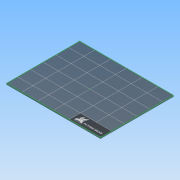
# Autodesk Inventor part: ультрабаза
Saved by Autodesk Inventor 2017 (Build 210142000, 142)
## iProperties
Part Number: ультрабаза
Material: Типовые
Document SubType Name: Modeling
Designer: Max
Mass: 234.623 g
Surface Area: 1209.8 cm^2
Volume: 234.623 cm^3
Density: 1 g/cm^3
Appearance: Металлическая сетка 01
Author: Max
Autodesk Inventor part; units mm, degrees
(part 1 of 2)
ref_plane "YZ Plane" through (0, 0, 0) normal (1, 0, 0) x (0, 1, 0)
ref_plane "XZ Plane" through (0, 0, 0) normal (0, 1, 0) x (-1, 0, 0)
ref_plane "XY Plane" through (0, 0, 0) normal (0, 0, 1) x (1, 0, 0)
sketch "Эскиз1" plane through (0, 0, 0) normal (0, 0, 1) x (1, 0, 0)
  line L0 (135.5, -107) -> (-135.5, -107)
  line L1 (-137.5, -105) -> (-137.5, 105)
  line L2 (-135.5, 107) -> (135.5, 107)
  line L3 (137.5, 105) -> (137.5, -105)
  line L4 (137.5, -107) -> (-137.5, 107) construction
  line L5 (-137.5, -107) -> (137.5, 107) construction
  arc A0 (-135.5, 107) -> (-137.5, 105) centre (-135.5, 105) ccw
  arc A1 (137.5, 105) -> (135.5, 107) centre (135.5, 105) ccw
  arc A2 (135.5, -107) -> (137.5, -105) centre (135.5, -105) ccw
  arc A3 (-137.5, -105) -> (-135.5, -107) centre (-135.5, -105) ccw
  point P0 (0, 0)
  dimension "d0" = 214
  dimension "d1" = 275
  dimension "d2" = 2
  constraints: 12 end point, 8 point on circle, 8 point on line, 8 tangent, 4 centre point, 3 equal radius, 2 midpoint, 2 parallel, 1 horizontal, 1 perpendicular
  measures "d0" distance between parallel lines of L0 L2
  measures "d1" distance between parallel lines of L3 L1
  measures "d2" radius of A0
extrude "Выдавливание1" add sketch "Эскиз1" along normal blind 4
chamfer "Фаска1" distance 1 angle 45 16 edges at (137.5, 0, 4) (136.9142, 106.4142, 4) (0, 107, 4) (-136.9142, 106.4142, 4) (-137.5, 0, 4) (-136.9142, -106.4142, 4) (0, -107, 4) (136.9142, -106.4142, 4) (137.5, 0, 0) (136.9142, 106.4142, 0) (0, 107, 0) (-136.9142, 106.4142, 0) (-137.5, 0, 0) (-136.9142, -106.4142, 0) (0, -107, 0) (136.9142, -106.4142, 0)
sketch "Эскиз2" plane through (0, 0, 4) normal (0, 0, 1) x (1, 0, 0)
  line L0 (136.5, 105) -> (136.5, -105) projected
  arc A0 (136.5, 105) -> (135.5, 106) centre (135.5, 105) ccw projected
  line L1 (-135.5, 106) -> (135.5, 106) projected
  arc A1 (-135.5, 106) -> (-136.5, 105) centre (-135.5, 105) ccw projected
  line L2 (-136.5, -105) -> (-136.5, 105) projected
  arc A2 (-136.5, -105) -> (-135.5, -106) centre (-135.5, -105) ccw projected
  line L3 (135.5, -106) -> (-135.5, -106) projected
  arc A3 (135.5, -106) -> (136.5, -105) centre (135.5, -105) ccw projected
  point P0 (0, 0)
sketch "Эскиз3" plane through (0, 0, 4) normal (0, 0, 1) x (1, 0, 0)
  line L0 (-136.5, -105) -> (-136.5, 105) projected
  line L1 (136.5, 105) -> (136.5, -105) projected
  line L2 (-136.5, 0.35) -> (136.5, 0.35)
  line L3 (136.5, 0.35) -> (136.5, -0.35)
  line L4 (136.5, -0.35) -> (-136.5, -0.35)
  line L5 (-136.5, -0.35) -> (-136.5, 0.35)
  line L6 (0, 0) -> (33.6599, 0) construction
  line L7 (0, 0) -> (0, 3.0622)
  line L8 (0, 3.0622) -> (0, 34.6111) construction
  line L9 (135.5, -106) -> (-135.5, -106) projected
  line L10 (-135.5, 106) -> (135.5, 106) projected
  line L11 (-0.35, -106) -> (0.35, -106)
  line L12 (0.35, -106) -> (0.35, 106)
  line L13 (0.35, 106) -> (-0.35, 106)
  line L14 (-0.35, 106) -> (-0.35, -106)
  dimension "d8" = 0.7
  dimension "d17" = 0.7
  constraints: 22 end point, 5 parallel, 5 point on line, 2 horizontal, 2 perpendicular, 2 other
  measures "d8" distance between parallel lines of L4 L2
  measures "d17" distance between parallel lines of L12 L14
extrude "Выдавливание2" add sketch "Эскиз3" along normal blind 0.1 contours L0 L2 L14 L4 | L14 L2 L12 L4 | L12 L2 L1 L4
pattern_linear "Прямоуг.массив1" count 3 spacing 37 along (0, 1, 0) count 3 spacing 37 along (0, -1, 0) of "Выдавливание2"
extrude "Выдавливание3" add sketch "Эскиз3" along normal blind 0.1 contours L14 L2 L12 L4 | L4 L12 L9 L14 | L14 L10 L12 L2
pattern_linear "Прямоуг.массив2" count 3 spacing 46 along (-1, 0, 0) count 3 spacing 46 along (1, 0, 0) of "Выдавливание3"
sketch "Эскиз4" plane through (0, 0, 4.1) normal (0, 0, 1) x (1, 0, 0)
  line L0 (-135.5, -106) -> (135.5, -106) projected
  line L1 (91.65, -74.35) -> (92.35, -74.35)
  line L2 (92.35, -74.35) -> (92.35, -106)
  line L3 (92.35, -106) -> (91.65, -106)
  line L4 (91.65, -106) -> (91.65, -74.35)
  line L5 (92.35, -106) -> (92.35, -74.35) projected
  point P0 (0, 0)
  constraints: 8 end point, 2 parallel, 1 collinear, 1 horizontal, 1 perpendicular, 1 point on line
extrude "Выдавливание4" cut sketch "Эскиз4" against normal blind 0.1
sketch "Эскиз6" plane through (0, 0, 4) normal (0, 0, 1) x (1, 0, 0)
  line L0 (47.8519, -76.7152) -> (78.2896, -76.7152) construction
  line L1 (78.2896, -76.7152) -> (78.2896, -107.153) construction
  line L2 (78.2896, -107.153) -> (47.8519, -107.153) construction
  line L3 (47.8519, -107.153) -> (47.8519, -76.7152) construction
  line L4 (58.0569, -84.1432) -> (58.585, -83.5976) construction
  line L5 (58.585, -83.5976) -> (59.2465, -82.9077) construction
  line L6 (59.2465, -82.9077) -> (59.6838, -82.432) construction
  line L7 (59.6838, -82.432) -> (59.9462, -82.0822) construction
  line L8 (59.9462, -82.0822) -> (60.5989, -81.4036) construction
  line L9 (60.5989, -81.4036) -> (61.1809, -80.7023) construction
  line L10 (61.1809, -80.7023) -> (61.3763, -80.4637) construction
  line L11 (61.3763, -80.4637) -> (62.6475, -78.5746) construction
  line L12 (62.6475, -78.5746) -> (62.8189, -78.3137) construction
  line L13 (62.8189, -78.3137) -> (63.1024, -77.7856) construction
  line L14 (63.1024, -77.7856) -> (63.3659, -77.2628) construction
  line L15 (63.3659, -77.2628) -> (63.6158, -76.7664) construction
  line L16 (63.6158, -76.7664) -> (63.6201, -76.7558) construction
  line L17 (63.6201, -76.7558) -> (63.6201, -76.7654) construction
  line L18 (63.6201, -76.7654) -> (63.7564, -77.0283) construction
  line L19 (63.7564, -77.0283) -> (64.02, -77.8831) construction
  line L20 (64.02, -77.8831) -> (64.0864, -78.3234) construction
  line L21 (64.0864, -78.3234) -> (64.0864, -78.7811) construction
  line L22 (64.0864, -78.7811) -> (63.9126, -80.1417) construction
  line L23 (63.9126, -80.1417) -> (63.6859, -80.7747) construction
  line L24 (63.6859, -80.7747) -> (63.2325, -81.8429) construction
  line L25 (63.2325, -81.8429) -> (62.816, -82.539) construction
  line L26 (62.816, -82.539) -> (62.3595, -83.2522) construction
  line L27 (62.3595, -83.2522) -> (62.2397, -83.4291) construction
  line L28 (62.2397, -83.4291) -> (62.0693, -83.676) construction
  line L29 (62.0693, -83.676) -> (62.1075, -83.6534) construction
  line L30 (62.1075, -83.6534) -> (62.1613, -83.6199) construction
  line L31 (62.1613, -83.6199) -> (62.3249, -83.4891) construction
  line L32 (62.3249, -83.4891) -> (62.9319, -82.8314) construction
  line L33 (62.9319, -82.8314) -> (63.8264, -81.7452) construction
  line L34 (63.8264, -81.7452) -> (64.8316, -80.3842) construction
  line L35 (64.8316, -80.3842) -> (64.8415, -80.3689) construction
  line L36 (64.8415, -80.3689) -> (64.836, -80.3846) construction
  line L37 (64.836, -80.3846) -> (64.8649, -80.4981) construction
  line L38 (64.8649, -80.4981) -> (64.9349, -80.9101) construction
  line L39 (64.9349, -80.9101) -> (65.0014, -81.5135) construction
  line L40 (65.0014, -81.5135) -> (64.9087, -82.4789) construction
  line L41 (64.9087, -82.4789) -> (64.606, -83.4734) construction
  line L42 (64.606, -83.4734) -> (64.1613, -84.3443) construction
  line L43 (64.1613, -84.3443) -> (63.6672, -85.1103) construction
  line L44 (63.6672, -85.1103) -> (62.9587, -85.9145) construction
  line L45 (62.9587, -85.9145) -> (62.6125, -86.2444) construction
  line L46 (62.6125, -86.2444) -> (62.3243, -86.521) construction
  line L47 (62.3243, -86.521) -> (62.171, -86.686) construction
  line L48 (62.171, -86.686) -> (62.162, -86.6995) construction
  line L49 (62.162, -86.6995) -> (62.1856, -86.6864) construction
  line L50 (62.1856, -86.6864) -> (62.4487, -86.5194) construction
  line L51 (62.4487, -86.5194) -> (62.7136, -86.3821) construction
  line L52 (62.7136, -86.3821) -> (63.2176, -86.0665) construction
  line L53 (63.2176, -86.0665) -> (63.723, -85.7352) construction
  line L54 (63.723, -85.7352) -> (64.0161, -85.4507) construction
  line L55 (64.0161, -85.4507) -> (64.3389, -85.1406) construction
  line L56 (64.3389, -85.1406) -> (64.5597, -84.9113) construction
  line L57 (64.5597, -84.9113) -> (64.5708, -84.896) construction
  line L58 (64.5708, -84.896) -> (64.5656, -84.9151) construction
  line L59 (64.5656, -84.9151) -> (64.6262, -85.2714) construction
  line L60 (64.6262, -85.2714) -> (64.5771, -85.7127) construction
  line L61 (64.5771, -85.7127) -> (64.1613, -87.1292) construction
  line L62 (64.1613, -87.1292) -> (63.5106, -88.2303) construction
  line L63 (63.5106, -88.2303) -> (62.3182, -89.6027) construction
  line L64 (62.3182, -89.6027) -> (62.3174, -89.6036) construction
  line L65 (62.3174, -89.6036) -> (62.32, -89.6029) construction
  line L66 (62.32, -89.6029) -> (62.9995, -89.5699) construction
  line L67 (62.9995, -89.5699) -> (63.0073, -89.5699) construction
  line L68 (63.0073, -89.5699) -> (63.0203, -89.5624) construction
  line L69 (63.0203, -89.5624) -> (63.3181, -89.4088) construction
  line L70 (63.3181, -89.4088) -> (63.7593, -89.0384) construction
  line L71 (63.7593, -89.0384) -> (64.1508, -88.6371) construction
  line L72 (64.1508, -88.6371) -> (64.5553, -88.1503) construction
  line L73 (64.5553, -88.1503) -> (64.9848, -87.3865) construction
  line L74 (64.9848, -87.3865) -> (65.1279, -86.9947) construction
  line L75 (65.1279, -86.9947) -> (65.3006, -86.2605) construction
  line L76 (65.3006, -86.2605) -> (65.3006, -85.8673) construction
  line L77 (65.3006, -85.8673) -> (65.3006, -85.207) construction
  line L78 (65.3006, -85.207) -> (65.1992, -84.7863) construction
  line L79 (65.1992, -84.7863) -> (65.0979, -84.5614) construction
  line L80 (65.0979, -84.5614) -> (64.9939, -84.3167) construction
  line L81 (64.9939, -84.3167) -> (64.9664, -84.1432) construction
  line L82 (64.9664, -84.1432) -> (64.9922, -83.8019) construction
  line L83 (64.9922, -83.8019) -> (65.1313, -83.509) construction
  line L84 (65.1313, -83.509) -> (65.3023, -83.2527) construction
  line L85 (65.3023, -83.2527) -> (65.74, -82.8881) construction
  line L86 (65.74, -82.8881) -> (66.2485, -82.5981) construction
  line L87 (66.2485, -82.5981) -> (67.1006, -82.2368) construction
  line L88 (67.1006, -82.2368) -> (68.0195, -81.8844) construction
  line L89 (68.0195, -81.8844) -> (69.5796, -81.1161) construction
  line L90 (69.5796, -81.1161) -> (71.2261, -80.3458) construction
  line L91 (71.2261, -80.3458) -> (72.7714, -79.4408) construction
  line L92 (72.7714, -79.4408) -> (73.5994, -78.8823) construction
  line L93 (73.5994, -78.8823) -> (75.316, -77.7088) construction
  line L94 (75.316, -77.7088) -> (75.8413, -77.2797) construction
  line L95 (75.8413, -77.2797) -> (76.1159, -77.0359) construction
  line L96 (76.1159, -77.0359) -> (76.2395, -76.9192) construction
  line L97 (76.2395, -76.9192) -> (76.2524, -76.9192) construction
  line L98 (76.2524, -76.9192) -> (76.2201, -77.0074) construction
  line L99 (76.2201, -77.0074) -> (76.2201, -77.2657) construction
  line L100 (76.2201, -77.2657) -> (76.1001, -77.9758) construction
  line L101 (76.1001, -77.9758) -> (75.8421, -78.9571) construction
  line L102 (75.8421, -78.9571) -> (75.5423, -79.5608) construction
  line L103 (75.5423, -79.5608) -> (75.0505, -80.2964) construction
  line L104 (75.0505, -80.2964) -> (74.6067, -80.8242) construction
  line L105 (74.6067, -80.8242) -> (73.3049, -82.0792) construction
  line L106 (73.3049, -82.0792) -> (72.4409, -82.7407) construction
  line L107 (72.4409, -82.7407) -> (71.1828, -83.5927) construction
  line L108 (71.1828, -83.5927) -> (70.7434, -83.8471) construction
  line L109 (70.7434, -83.8471) -> (70.7434, -83.8614) construction
  line L110 (70.7434, -83.8614) -> (70.8232, -83.9129) construction
  line L111 (70.8232, -83.9129) -> (70.9595, -83.8861) construction
  line L112 (70.9595, -83.8861) -> (71.9932, -83.4155) construction
  line L113 (71.9932, -83.4155) -> (73.7755, -82.4723) construction
  line L114 (73.7755, -82.4723) -> (74.7969, -81.873) construction
  line L115 (74.7969, -81.873) -> (75.4744, -81.4665) construction
  line L116 (75.4744, -81.4665) -> (75.4973, -81.4518) construction
  line L117 (75.4973, -81.4518) -> (75.4973, -81.5379) construction
  line L118 (75.4973, -81.5379) -> (75.2536, -82.3724) construction
  line L119 (75.2536, -82.3724) -> (74.3062, -83.9127) construction
  line L120 (74.3062, -83.9127) -> (73.7236, -84.5338) construction
  line L121 (73.7236, -84.5338) -> (72.7954, -85.3581) construction
  line L122 (72.7954, -85.3581) -> (72.0406, -85.8668) construction
  line L123 (72.0406, -85.8668) -> (71.0807, -86.4494) construction
  line L124 (71.0807, -86.4494) -> (70.1289, -86.8842) construction
  line L125 (70.1289, -86.8842) -> (69.3987, -87.2042) construction
  line L126 (69.3987, -87.2042) -> (69.1115, -87.2616) construction
  line L127 (69.1115, -87.2616) -> (69.0889, -87.306) construction
  line L128 (69.0889, -87.306) -> (69.1488, -87.3298) construction
  line L129 (69.1488, -87.3298) -> (70.1619, -87.2655) construction
  line L130 (70.1619, -87.2655) -> (71.1536, -87.0008) construction
  line L131 (71.1536, -87.0008) -> (71.7613, -86.7659) construction
  line L132 (71.7613, -86.7659) -> (72.5321, -86.4474) construction
  line L133 (72.5321, -86.4474) -> (72.6124, -86.4147) construction
  line L134 (72.6124, -86.4147) -> (72.5643, -86.4496) construction
  line L135 (72.5643, -86.4496) -> (72.4297, -86.7091) construction
  line L136 (72.4297, -86.7091) -> (72.0429, -87.336) construction
  line L137 (72.0429, -87.336) -> (71.7462, -87.7207) construction
  line L138 (71.7462, -87.7207) -> (71.1519, -88.3518) construction
  line L139 (71.1519, -88.3518) -> (70.3788, -89.0405) construction
  line L140 (70.3788, -89.0405) -> (69.6666, -89.4997) construction
  line L141 (69.6666, -89.4997) -> (68.9778, -89.9073) construction
  line L142 (68.9778, -89.9073) -> (68.7389, -90.0573) construction
  line L143 (68.7389, -90.0573) -> (68.7212, -90.0868) construction
  line L144 (68.7212, -90.0868) -> (68.9979, -90.0868) construction
  line L145 (68.9979, -90.0868) -> (69.6455, -90.1548) construction
  line L146 (69.6455, -90.1548) -> (70.6365, -90.3216) construction
  line L147 (70.6365, -90.3216) -> (70.8988, -90.3216) construction
  line L148 (70.8988, -90.3216) -> (72.8573, -91.6694) construction
  line L149 (72.8573, -91.6694) -> (72.8654, -91.6787) construction
  line L150 (72.8654, -91.6787) -> (72.8941, -91.7359) construction
  line L151 (72.8941, -91.7359) -> (73.23, -92.4126) construction
  line L152 (73.23, -92.4126) -> (73.23, -92.496) construction
  line L153 (73.23, -92.496) -> (73.163, -92.7094) construction
  line L154 (73.163, -92.7094) -> (73.0011, -93.1785) construction
  line L155 (73.0011, -93.1785) -> (72.8815, -93.3901) construction
  line L156 (72.8815, -93.3901) -> (72.83, -93.403) construction
  line L157 (72.83, -93.403) -> (72.83, -93.3828) construction
  line L158 (72.83, -93.3828) -> (72.83, -93.3036) construction
  line L159 (72.83, -93.3036) -> (72.8116, -93.0902) construction
  line L160 (72.8116, -93.0902) -> (72.7674, -92.8952) construction
  line L161 (72.7674, -92.8952) -> (72.6515, -92.577) construction
  line L162 (72.6515, -92.577) -> (72.3701, -92.3194) construction
  line L163 (72.3701, -92.3194) -> (72.1033, -92.0876) construction
  line L164 (72.1033, -92.0876) -> (71.9782, -92.0379) construction
  line L165 (71.9782, -92.0379) -> (71.9285, -92.025) construction
  line L166 (71.9285, -92.025) -> (71.946, -92.0337) construction
  line L167 (71.946, -92.0337) -> (72.0417, -92.1122) construction
  line L168 (72.0417, -92.1122) -> (72.2698, -92.3774) construction
  line L169 (72.2698, -92.3774) -> (72.5703, -92.7673) construction
  line L170 (72.5703, -92.7673) -> (72.6719, -93.0395) construction
  line L171 (72.6719, -93.0395) -> (72.7693, -93.4294) construction
  line L172 (72.7693, -93.4294) -> (72.7693, -93.5984) construction
  line L173 (72.7693, -93.5984) -> (72.7693, -94.6006) construction
  line L174 (72.7693, -94.6006) -> (72.7693, -94.721) construction
  line L175 (72.7693, -94.721) -> (73.012, -95.0062) construction
  line L176 (73.012, -95.0062) -> (73.6685, -95.948) construction
  line L177 (73.6685, -95.948) -> (73.7068, -96.0386) construction
  line L178 (73.7068, -96.0386) -> (73.7068, -96.2499) construction
  line L179 (73.7068, -96.2499) -> (74.0406, -97.4838) construction
  line L180 (74.0406, -97.4838) -> (74.0406, -97.6417) construction
  line L181 (74.0406, -97.6417) -> (74.0046, -97.9554) construction
  line L182 (74.0046, -97.9554) -> (73.7015, -99.536) construction
  line L183 (73.7015, -99.536) -> (73.673, -99.536) construction
  line L184 (73.673, -99.536) -> (73.5426, -99.536) construction
  line L185 (73.5426, -99.536) -> (72.5119, -99.536) construction
  line L186 (72.5119, -99.536) -> (72.4208, -99.536) construction
  line L187 (72.4208, -99.536) -> (72.2665, -99.2589) construction
  line L188 (72.2665, -99.2589) -> (71.6001, -98.5264) construction
  line L189 (71.6001, -98.5264) -> (71.4238, -98.2675) construction
  line L190 (71.4238, -98.2675) -> (70.4213, -96.7197) construction
  line L191 (70.4213, -96.7197) -> (70.3885, -96.6426) construction
  line L192 (70.3885, -96.6426) -> (70.3113, -96.6216) construction
  line L193 (70.3113, -96.6216) -> (67.9932, -95.6736) construction
  line L194 (67.9932, -95.6736) -> (67.977, -95.6736) construction
  line L195 (67.977, -95.6736) -> (67.977, -95.7933) construction
  line L196 (67.977, -95.7933) -> (70.1244, -96.8272) construction
  line L197 (70.1244, -96.8272) -> (70.2246, -96.9143) construction
  line L198 (70.2246, -96.9143) -> (70.4218, -97.1682) construction
  line L199 (70.4218, -97.1682) -> (71.2221, -98.1928) construction
  line L200 (71.2221, -98.1928) -> (71.4717, -98.5349) construction
  line L201 (71.4717, -98.5349) -> (71.4717, -98.7274) construction
  line L202 (71.4717, -98.7274) -> (71.1015, -98.9495) construction
  line L203 (71.1015, -98.9495) -> (70.8349, -98.9495) construction
  line L204 (70.8349, -98.9495) -> (70.1833, -98.7669) construction
  line L205 (70.1833, -98.7669) -> (69.2694, -98.5446) construction
  line L206 (69.2694, -98.5446) -> (68.5464, -98.0323) construction
  line L207 (68.5464, -98.0323) -> (67.1489, -97.0367) construction
  line L208 (67.1489, -97.0367) -> (66.0385, -96.137) construction
  line L209 (66.0385, -96.137) -> (66.07, -96.1214) construction
  line L210 (66.07, -96.1214) -> (65.9547, -96.2124) construction
  line L211 (65.9547, -96.2124) -> (64.6537, -96.8644) construction
  line L212 (64.6537, -96.8644) -> (64.5984, -96.8644) construction
  line L213 (64.5984, -96.8644) -> (64.3032, -96.8644) construction
  line L214 (64.3032, -96.8644) -> (62.2656, -96.8644) construction
  line L215 (62.2656, -96.8644) -> (62.2288, -96.8561) construction
  line L216 (62.2288, -96.8561) -> (62.1845, -96.8167) construction
  line L217 (62.1845, -96.8167) -> (60.8689, -96.2809) construction
  line L218 (60.8689, -96.2809) -> (60.8266, -96.2809) construction
  line L219 (60.8266, -96.2809) -> (60.6629, -96.4775) construction
  line L220 (60.6629, -96.4775) -> (58.7049, -98.0118) construction
  line L221 (58.7049, -98.0118) -> (58.6154, -98.0651) construction
  line L222 (58.6154, -98.0651) -> (57.6146, -98.3598) construction
  line L223 (57.6146, -98.3598) -> (56.0021, -98.9381) construction
  line L224 (56.0021, -98.9381) -> (55.7852, -98.9715) construction
  line L225 (55.7852, -98.9715) -> (55.4405, -98.8492) construction
  line L226 (55.4405, -98.8492) -> (55.0624, -98.6823) construction
  line L227 (55.0624, -98.6823) -> (55.0624, -98.6656) construction
  line L228 (55.0624, -98.6656) -> (55.1681, -98.6088) construction
  line L229 (55.1681, -98.6088) -> (56.837, -97.1126) construction
  line L230 (56.837, -97.1126) -> (56.8672, -97.0916) construction
  line L231 (56.8672, -97.0916) -> (56.9191, -96.9557) construction
  line L232 (56.9191, -96.9557) -> (57.4616, -96.0024) construction
  line L233 (57.4616, -96.0024) -> (57.4616, -95.9863) construction
  line L234 (57.4616, -95.9863) -> (57.2446, -95.8979) construction
  line L235 (57.2446, -95.8979) -> (57.1964, -95.9519) construction
  line L236 (57.1964, -95.9519) -> (56.6746, -97.0084) construction
  line L237 (56.6746, -97.0084) -> (56.6189, -97.0976) construction
  line L238 (56.6189, -97.0976) -> (54.7059, -98.7912) construction
  line L239 (54.7059, -98.7912) -> (54.588, -98.8386) construction
  line L240 (54.588, -98.8386) -> (54.1498, -98.8386) construction
  line L241 (54.1498, -98.8386) -> (53.7434, -98.7814) construction
  line L242 (53.7434, -98.7814) -> (53.1643, -98.6693) construction
  line L243 (53.1643, -98.6693) -> (52.9154, -98.3774) construction
  line L244 (52.9154, -98.3774) -> (52.9154, -98.2185) construction
  line L245 (52.9154, -98.2185) -> (53.0184, -98.0297) construction
  line L246 (53.0184, -98.0297) -> (53.4219, -97.7635) construction
  line L247 (53.4219, -97.7635) -> (53.7439, -97.6862) construction
  line L248 (53.7439, -97.6862) -> (54.1302, -97.4544) construction
  line L249 (54.1302, -97.4544) -> (54.186, -97.3943) construction
  line L250 (54.186, -97.3943) -> (54.4135, -97.1024) construction
  line L251 (54.4135, -97.1024) -> (54.4994, -96.8105) construction
  line L252 (54.4994, -96.8105) -> (54.5401, -96.6496) construction
  line L253 (54.5401, -96.6496) -> (54.488, -96.3832) construction
  line L254 (54.488, -96.3832) -> (54.4605, -96.3832) construction
  line L255 (54.4605, -96.3832) -> (54.2952, -96.4353) construction
  line L256 (54.2952, -96.4353) -> (53.9615, -96.5516) construction
  line L257 (53.9615, -96.5516) -> (53.4319, -96.6771) construction
  line L258 (53.4319, -96.6771) -> (52.9313, -96.6428) construction
  line L259 (52.9313, -96.6428) -> (52.2167, -96.586) construction
  line L260 (52.2167, -96.586) -> (52.0436, -96.5378) construction
  line L261 (52.0436, -96.5378) -> (51.6736, -96.4078) construction
  line L262 (51.6736, -96.4078) -> (51.2587, -96.0429) construction
  line L263 (51.2587, -96.0429) -> (51.2187, -95.8179) construction
  line L264 (51.2187, -95.8179) -> (51.2187, -95.468) construction
  line L265 (51.2187, -95.468) -> (51.4037, -95.143) construction
  line L266 (51.4037, -95.143) -> (51.6679, -94.9102) construction
  line L267 (51.6679, -94.9102) -> (52.0023, -94.5884) construction
  line L268 (52.0023, -94.5884) -> (52.1712, -94.4579) construction
  line L269 (52.1712, -94.4579) -> (52.3962, -93.9588) construction
  line L270 (52.3962, -93.9588) -> (52.5081, -93.6574) construction
  line L271 (52.5081, -93.6574) -> (52.7708, -93.4119) construction
  line L272 (52.7708, -93.4119) -> (52.958, -93.2339) construction
  line L273 (52.958, -93.2339) -> (52.9955, -93.115) construction
  line L274 (52.9955, -93.115) -> (52.969, -92.6609) construction
  line L275 (52.969, -92.6609) -> (53.0022, -92.4995) construction
  line L276 (53.0022, -92.4995) -> (53.0928, -92.2897) construction
  line L277 (53.0928, -92.2897) -> (53.2466, -92.1002) construction
  line L278 (53.2466, -92.1002) -> (53.311, -92.0108) construction
  line L279 (53.311, -92.0108) -> (53.6436, -92.0537) construction
  line L280 (53.6436, -92.0537) -> (53.8046, -92.2111) construction
  line L281 (53.8046, -92.2111) -> (53.8689, -92.372) construction
  line L282 (53.8689, -92.372) -> (53.8689, -92.4614) construction
  line L283 (53.8689, -92.4614) -> (53.966, -92.4614) construction
  line L284 (53.966, -92.4614) -> (54.0916, -92.3879) construction
  line L285 (54.0916, -92.3879) -> (54.2144, -92.2937) construction
  line L286 (54.2144, -92.2937) -> (54.2747, -92.0589) construction
  line L287 (54.2747, -92.0589) -> (55.1161, -91.3179) construction
  line L288 (55.1161, -91.3179) -> (55.2203, -91.2446) construction
  line L289 (55.2203, -91.2446) -> (55.448, -91.2021) construction
  line L290 (55.448, -91.2021) -> (56.0672, -90.9846) construction
  line L291 (56.0672, -90.9846) -> (56.3968, -90.8613) construction
  line L292 (56.3968, -90.8613) -> (56.4923, -90.8305) construction
  line L293 (56.4923, -90.8305) -> (56.4923, -90.8476) construction
  line L294 (56.4923, -90.8476) -> (57.8422, -90.8476) construction
  line L295 (57.8422, -90.8476) -> (57.8546, -90.8623) construction
  line L296 (57.8546, -90.8623) -> (57.9562, -91.0106) construction
  line L297 (57.9562, -91.0106) -> (58.2231, -91.3707) construction
  line L298 (58.2231, -91.3707) -> (58.2717, -91.3896) construction
  line L299 (58.2717, -91.3896) -> (58.3207, -91.3642) construction
  line L300 (58.3207, -91.3642) -> (58.3106, -91.3541) construction
  line L301 (58.3106, -91.3541) -> (58.3106, -91.2256) construction
  line L302 (58.3106, -91.2256) -> (57.9876, -90.7386) construction
  line L303 (57.9876, -90.7386) -> (57.9741, -90.7386) construction
  line L304 (57.9741, -90.7386) -> (57.8676, -90.7487) construction
  line L305 (57.8676, -90.7487) -> (56.6643, -90.7487) construction
  line L306 (56.6643, -90.7487) -> (56.6695, -90.7443) construction
  line L307 (56.6695, -90.7443) -> (56.7055, -90.7402) construction
  line L308 (56.7055, -90.7402) -> (56.9153, -90.6986) construction
  line L309 (56.9153, -90.6986) -> (57.278, -90.5923) construction
  line L310 (57.278, -90.5923) -> (57.9008, -90.2282) construction
  line L311 (57.9008, -90.2282) -> (58.0094, -90.1738) construction
  line L312 (58.0094, -90.1738) -> (58.1797, -90.1895) construction
  line L313 (58.1797, -90.1895) -> (58.4019, -90.1845) construction
  line L314 (58.4019, -90.1845) -> (58.4906, -90.1522) construction
  line L315 (58.4906, -90.1522) -> (58.6554, -90.0119) construction
  line L316 (58.6554, -90.0119) -> (58.8609, -89.6211) construction
  line L317 (58.8609, -89.6211) -> (59.0588, -89.2185) construction
  line L318 (59.0588, -89.2185) -> (59.1508, -88.7991) construction
  line L319 (59.1508, -88.7991) -> (59.1881, -88.5779) construction
  line L320 (59.1881, -88.5779) -> (59.2722, -88.0098) construction
  line L321 (59.2722, -88.0098) -> (59.1722, -87.2811) construction
  line L322 (59.1722, -87.2811) -> (58.9901, -86.7345) construction
  line L323 (58.9901, -86.7345) -> (58.7961, -86.3466) construction
  line L324 (58.7961, -86.3466) -> (58.4788, -85.8882) construction
  line L325 (58.4788, -85.8882) -> (58.1908, -85.6297) construction
  line L326 (58.1908, -85.6297) -> (57.9841, -85.3958) construction
  line L327 (57.9841, -85.3958) -> (57.8643, -85.1375) construction
  line L328 (57.8643, -85.1375) -> (57.8194, -84.8679) construction
  line L329 (57.8194, -84.8679) -> (57.8531, -84.6057) construction
  line L330 (57.8531, -84.6057) -> (57.9055, -84.3548) construction
  line L331 (57.9055, -84.3548) -> (57.9804, -84.235) construction
  line L332 (57.9804, -84.235) -> (58.0569, -84.1432) construction
  spline S0 degree 4 poles (58.0569, -84.1432) (58.585, -83.5976) (59.2465, -82.9077) (59.6838, -82.432) (59.9462, -82.0822) (60.5989, -81.4036) (61.1809, -80.7023) (61.3763, -80.4637) (62.6475, -78.5746) (62.8189, -78.3137) (63.1024, -77.7856) (63.3659, -77.2628) (63.6158, -76.7664) (63.6201, -76.7558) (63.6201, -76.7654) (63.7564, -77.0283) (64.02, -77.8831) (64.0864, -78.3234) (64.0864, -78.7811) (63.9126, -80.1417) (63.6859, -80.7747) (63.2325, -81.8429) (62.816, -82.539) (62.3595, -83.2522) (62.2397, -83.4291) (62.0693, -83.676) (62.1075, -83.6534) (62.1613, -83.6199) (62.3249, -83.4891) (62.9319, -82.8314) (63.8264, -81.7452) (64.8316, -80.3842) (64.8415, -80.3689) (64.836, -80.3846) (64.8649, -80.4981) (64.9349, -80.9101) (65.0014, -81.5135) (64.9087, -82.4789) (64.606, -83.4734) (64.1613, -84.3443) (63.6672, -85.1103) (62.9587, -85.9145) (62.6125, -86.2444) (62.3243, -86.521) (62.171, -86.686) (62.162, -86.6995) (62.1856, -86.6864) (62.4487, -86.5194) (62.7136, -86.3821) (63.2176, -86.0665) (63.723, -85.7352) (64.0161, -85.4507) (64.3389, -85.1406) (64.5597, -84.9113) (64.5708, -84.896) (64.5656, -84.9151) (64.6262, -85.2714) (64.5771, -85.7127) (64.1613, -87.1292) (63.5106, -88.2303) (62.3182, -89.6027) (62.3174, -89.6036) (62.32, -89.6029) (62.9995, -89.5699) (63.0073, -89.5699) (63.0203, -89.5624) (63.3181, -89.4088) (63.7593, -89.0384) (64.1508, -88.6371) (64.5553, -88.1503) (64.9848, -87.3865) (65.1279, -86.9947) (65.3006, -86.2605) (65.3006, -85.8673) (65.3006, -85.207) (65.1992, -84.7863) (65.0979, -84.5614) (64.9939, -84.3167) (64.9664, -84.1432) (64.9922, -83.8019) (65.1313, -83.509) (65.3023, -83.2527) (65.74, -82.8881) (66.2485, -82.5981) (67.1006, -82.2368) (68.0195, -81.8844) (69.5796, -81.1161) (71.2261, -80.3458) (72.7714, -79.4408) (73.5994, -78.8823) (75.316, -77.7088) (75.8413, -77.2797) (76.1159, -77.0359) (76.2395, -76.9192) (76.2524, -76.9192) (76.2201, -77.0074) (76.2201, -77.2657) (76.1001, -77.9758) (75.8421, -78.9571) (75.5423, -79.5608) (75.0505, -80.2964) (74.6067, -80.8242) (73.3049, -82.0792) (72.4409, -82.7407) (71.1828, -83.5927) (70.7434, -83.8471) (70.7434, -83.8614) (70.8232, -83.9129) (70.9595, -83.8861) (71.9932, -83.4155) (73.7755, -82.4723) (74.7969, -81.873) (75.4744, -81.4665) (75.4973, -81.4518) (75.4973, -81.5379) (75.2536, -82.3724) (74.3062, -83.9127) (73.7236, -84.5338) (72.7954, -85.3581) (72.0406, -85.8668) (71.0807, -86.4494) (70.1289, -86.8842) (69.3987, -87.2042) (69.1115, -87.2616) (69.0889, -87.306) (69.1488, -87.3298) (70.1619, -87.2655) (71.1536, -87.0008) (71.7613, -86.7659) (72.5321, -86.4474) (72.6124, -86.4147) (72.5643, -86.4496) (72.4297, -86.7091) (72.0429, -87.336) (71.7462, -87.7207) (71.1519, -88.3518) (70.3788, -89.0405) (69.6666, -89.4997) (68.9778, -89.9073) (68.7389, -90.0573) (68.7212, -90.0868) (68.9979, -90.0868) (69.6455, -90.1548) (70.6365, -90.3216) (70.8988, -90.3216) (72.8573, -91.6694) (72.8654, -91.6787) (72.8941, -91.7359) (73.23, -92.4126) (73.23, -92.496) (73.163, -92.7094) (73.0011, -93.1785) (72.8815, -93.3901) (72.83, -93.403) (72.83, -93.3828) (72.83, -93.3036) (72.8116, -93.0902) (72.7674, -92.8952) (72.6515, -92.577) (72.3701, -92.3194) (72.1033, -92.0876) (71.9782, -92.0379) (71.9285, -92.025) (71.946, -92.0337) (72.0417, -92.1122) (72.2698, -92.3774) (72.5703, -92.7673) (72.6719, -93.0395) (72.7693, -93.4294) (72.7693, -93.5984) (72.7693, -94.6006) (72.7693, -94.721) (73.012, -95.0062) (73.6685, -95.948) (73.7068, -96.0386) (73.7068, -96.2499) (74.0406, -97.4838) (74.0406, -97.6417) (74.0046, -97.9554) (73.7015, -99.536) (73.673, -99.536) (73.5426, -99.536) (72.5119, -99.536) (72.4208, -99.536) (72.2665, -99.2589) (71.6001, -98.5264) (71.4238, -98.2675) (70.4213, -96.7197) (70.3885, -96.6426) (70.3113, -96.6216) (67.9932, -95.6736) (67.977, -95.6736) (67.977, -95.7933) (70.1244, -96.8272) (70.2246, -96.9143) (70.4218, -97.1682) (71.2221, -98.1928) (71.4717, -98.5349) (71.4717, -98.7274) (71.1015, -98.9495) (70.8349, -98.9495) (70.1833, -98.7669) (69.2694, -98.5446) (68.5464, -98.0323) (67.1489, -97.0367) (66.0385, -96.137) (66.07, -96.1214) (65.9547, -96.2124) (64.6537, -96.8644) (64.5984, -96.8644) (64.3032, -96.8644) (62.2656, -96.8644) (62.2288, -96.8561) (62.1845, -96.8167) (60.8689, -96.2809) (60.8266, -96.2809) (60.6629, -96.4775) (58.7049, -98.0118) (58.6154, -98.0651) (57.6146, -98.3598) (56.0021, -98.9381) (55.7852, -98.9715) (55.4405, -98.8492) (55.0624, -98.6823) (55.0624, -98.6656) (55.1681, -98.6088) (56.837, -97.1126) (56.8672, -97.0916) (56.9191, -96.9557) (57.4616, -96.0024) (57.4616, -95.9863) (57.2446, -95.8979) (57.1964, -95.9519) (56.6746, -97.0084) (56.6189, -97.0976) (54.7059, -98.7912) (54.588, -98.8386) (54.1498, -98.8386) (53.7434, -98.7814) (53.1643, -98.6693) (52.9154, -98.3774) (52.9154, -98.2185) (53.0184, -98.0297) (53.4219, -97.7635) (53.7439, -97.6862) (54.1302, -97.4544) (54.186, -97.3943) (54.4135, -97.1024) (54.4994, -96.8105) (54.5401, -96.6496) (54.488, -96.3832) (54.4605, -96.3832) (54.2952, -96.4353) (53.9615, -96.5516) (53.4319, -96.6771) (52.9313, -96.6428) (52.2167, -96.586) (52.0436, -96.5378) (51.6736, -96.4078) (51.2587, -96.0429) (51.2187, -95.8179) (51.2187, -95.468) (51.4037, -95.143) (51.6679, -94.9102) (52.0023, -94.5884) (52.1712, -94.4579) (52.3962, -93.9588) (52.5081, -93.6574) (52.7708, -93.4119) (52.958, -93.2339) (52.9955, -93.115) (52.969, -92.6609) (53.0022, -92.4995) (53.0928, -92.2897) (53.2466, -92.1002) (53.311, -92.0108) (53.6436, -92.0537) (53.8046, -92.2111) (53.8689, -92.372) (53.8689, -92.4614) (53.966, -92.4614) (54.0916, -92.3879) (54.2144, -92.2937) (54.2747, -92.0589) (55.1161, -91.3179) (55.2203, -91.2446) (55.448, -91.2021) (56.0672, -90.9846) (56.3968, -90.8613) (56.4923, -90.8305) (56.4923, -90.8476) (57.8422, -90.8476) (57.8546, -90.8623) (57.9562, -91.0106) (58.2231, -91.3707) (58.2717, -91.3896) (58.3207, -91.3642) (58.3106, -91.3541) (58.3106, -91.2256) (57.9876, -90.7386) (57.9741, -90.7386) (57.8676, -90.7487) (56.6643, -90.7487) (56.6695, -90.7443) (56.7055, -90.7402) (56.9153, -90.6986) (57.278, -90.5923) (57.9008, -90.2282) (58.0094, -90.1738) (58.1797, -90.1895) (58.4019, -90.1845) (58.4906, -90.1522) (58.6554, -90.0119) (58.8609, -89.6211) (59.0588, -89.2185) (59.1508, -88.7991) (59.1881, -88.5779) (59.2722, -88.0098) (59.1722, -87.2811) (58.9901, -86.7345) (58.7961, -86.3466) (58.4788, -85.8882) (58.1908, -85.6297) (57.9841, -85.3958) (57.8643, -85.1375) (57.8194, -84.8679) (57.8531, -84.6057) (57.9055, -84.3548) (57.9804, -84.235) (58.0569, -84.1432) knots 1 1 1 1 1 2 3 4 5 6 7 8 9 10 11 12 13 14 15 16 17 18 19 20 21 22 23 24 25 26 27 28 29 30 31 32 33 34 35 36 37 38 39 40 41 42 43 44 45 46 47 48 49 50 51 52 53 54 55 56 57 58 59 60 61 62 63 64 65 66 67 68 69 70 71 72 73 74 75 76 77 78 79 80 81 82 83 84 85 86 87 88 89 90 91 92 93 94 95 96 97 98 99 100 101 102 103 104 105 106 107 108 109 110 111 112 113 114 115 116 117 118 119 120 121 122 123 124 125 126 127 128 129 130 131 132 133 134 135 136 137 138 139 140 141 142 143 144 145 146 147 148 149 150 151 152 153 154 155 156 157 158 159 160 161 162 163 164 165 166 167 168 169 170 171 172 173 174 175 176 177 178 179 180 181 182 183 184 185 186 187 188 189 190 191 192 193 194 195 196 197 198 199 200 201 202 203 204 205 206 207 208 209 210 211 212 213 214 215 216 217 218 219 220 221 222 223 224 225 226 227 228 229 230 231 232 233 234 235 236 237 238 239 240 241 242 243 244 245 246 247 248 249 250 251 252 253 254 255 256 257 258 259 260 261 262 263 264 265 266 267 268 269 270 271 272 273 274 275 276 277 278 279 280 281 282 283 284 285 286 287 288 289 290 291 292 293 294 295 296 297 298 299 300 301 302 303 304 305 306 307 308 309 310 311 312 313 314 315 316 317 318 319 320 321 322 323 324 325 326 327 327 327 327 327
  line L333 (55.426, -92.7574) -> (55.6687, -92.582) construction
  line L334 (55.6687, -92.582) -> (55.8986, -92.5002) construction
  line L335 (55.8986, -92.5002) -> (56.0194, -92.4222) construction
  line L336 (56.0194, -92.4222) -> (56.0633, -92.4327) construction
  line L337 (56.0633, -92.4327) -> (56.0945, -92.5246) construction
  line L338 (56.0945, -92.5246) -> (56.2372, -92.7231) construction
  line L339 (56.2372, -92.7231) -> (56.2864, -92.8691) construction
  line L340 (56.2864, -92.8691) -> (56.3012, -92.9413) construction
  line L341 (56.3012, -92.9413) -> (56.2454, -92.9413) construction
  line L342 (56.2454, -92.9413) -> (56.042, -92.9413) construction
  line L343 (56.042, -92.9413) -> (55.9829, -92.9413) construction
  line L344 (55.9829, -92.9413) -> (55.9961, -92.8445) construction
  line L345 (55.9961, -92.8445) -> (55.9846, -92.7574) construction
  line L346 (55.9846, -92.7574) -> (55.9436, -92.6706) construction
  line L347 (55.9436, -92.6706) -> (55.8632, -92.6706) construction
  line L348 (55.8632, -92.6706) -> (55.6696, -92.6985) construction
  line L349 (55.6696, -92.6985) -> (55.5088, -92.7904) construction
  line L350 (55.5088, -92.7904) -> (55.4465, -92.8183) construction
  line L351 (55.4465, -92.8183) -> (55.426, -92.7789) construction
  line L352 (55.426, -92.7789) -> (55.426, -92.7574) construction
  spline S1 degree 4 poles (55.426, -92.7574) (55.6687, -92.582) (55.8986, -92.5002) (56.0194, -92.4222) (56.0633, -92.4327) (56.0945, -92.5246) (56.2372, -92.7231) (56.2864, -92.8691) (56.3012, -92.9413) (56.2454, -92.9413) (56.042, -92.9413) (55.9829, -92.9413) (55.9961, -92.8445) (55.9846, -92.7574) (55.9436, -92.6706) (55.8632, -92.6706) (55.6696, -92.6985) (55.5088, -92.7904) (55.4465, -92.8183) (55.426, -92.7789) (55.426, -92.7574) knots 1 1 1 1 1 2 3 4 5 6 7 8 9 10 11 12 13 14 15 16 17 18 18 18 18 18
  line L353 (53.1142, -92.7574) -> (53.2687, -92.4663) construction
  line L354 (53.2687, -92.4663) -> (53.3183, -92.3098) construction
  line L355 (53.3183, -92.3098) -> (53.3619, -92.2721) construction
  line L356 (53.3619, -92.2721) -> (53.5548, -92.3521) construction
  line L357 (53.5548, -92.3521) -> (53.624, -92.4553) construction
  line L358 (53.624, -92.4553) -> (53.7555, -92.4864) construction
  line L359 (53.7555, -92.4864) -> (53.7555, -92.5203) construction
  line L360 (53.7555, -92.5203) -> (53.6989, -92.5697) construction
  line L361 (53.6989, -92.5697) -> (53.5689, -92.6362) construction
  line L362 (53.5689, -92.6362) -> (53.5053, -92.6687) construction
  line L363 (53.5053, -92.6687) -> (53.4898, -92.6206) construction
  line L364 (53.4898, -92.6206) -> (53.5068, -92.5485) construction
  line L365 (53.5068, -92.5485) -> (53.4742, -92.485) construction
  line L366 (53.4742, -92.485) -> (53.4092, -92.4722) construction
  line L367 (53.4092, -92.4722) -> (53.3442, -92.5627) construction
  line L368 (53.3442, -92.5627) -> (53.2538, -92.68) construction
  line L369 (53.2538, -92.68) -> (53.2043, -92.745) construction
  line L370 (53.2043, -92.745) -> (53.1747, -92.7987) construction
  line L371 (53.1747, -92.7987) -> (53.1266, -92.7987) construction
  line L372 (53.1266, -92.7987) -> (53.1142, -92.7574) construction
  spline S2 degree 4 poles (53.1142, -92.7574) (53.2687, -92.4663) (53.3183, -92.3098) (53.3619, -92.2721) (53.5548, -92.3521) (53.624, -92.4553) (53.7555, -92.4864) (53.7555, -92.5203) (53.6989, -92.5697) (53.5689, -92.6362) (53.5053, -92.6687) (53.4898, -92.6206) (53.5068, -92.5485) (53.4742, -92.485) (53.4092, -92.4722) (53.3442, -92.5627) (53.2538, -92.68) (53.2043, -92.745) (53.1747, -92.7987) (53.1266, -92.7987) (53.1142, -92.7574) knots 1 1 1 1 1 2 3 4 5 6 7 8 9 10 11 12 13 14 15 16 17 18 18 18 18 18
  line L373 (53.1363, -93.5716) -> (53.0988, -93.4618) construction
  line L374 (53.0988, -93.4618) -> (53.0207, -93.4126) construction
  line L375 (53.0207, -93.4126) -> (52.9369, -93.4762) construction
  line L376 (52.9369, -93.4762) -> (52.8039, -93.6352) construction
  line L377 (52.8039, -93.6352) -> (52.6092, -93.9366) construction
  line L378 (52.6092, -93.9366) -> (52.4824, -94.2341) construction
  line L379 (52.4824, -94.2341) -> (52.3511, -94.4615) construction
  line L380 (52.3511, -94.4615) -> (52.1762, -94.6759) construction
  line L381 (52.1762, -94.6759) -> (51.9637, -94.861) construction
  line L382 (51.9637, -94.861) -> (51.6855, -95.0876) construction
  line L383 (51.6855, -95.0876) -> (51.4504, -95.3858) construction
  line L384 (51.4504, -95.3858) -> (51.3749, -95.5766) construction
  line L385 (51.3749, -95.5766) -> (51.3749, -95.7118) construction
  line L386 (51.3749, -95.7118) -> (51.3967, -95.8767) construction
  line L387 (51.3967, -95.8767) -> (51.6012, -96.1247) construction
  line L388 (51.6012, -96.1247) -> (51.9532, -96.3155) construction
  line L389 (51.9532, -96.3155) -> (52.3429, -96.4499) construction
  line L390 (52.3429, -96.4499) -> (52.9798, -96.4714) construction
  line L391 (52.9798, -96.4714) -> (53.3775, -96.4956) construction
  line L392 (53.3775, -96.4956) -> (53.7995, -96.4015) construction
  line L393 (53.7995, -96.4015) -> (54.2644, -96.2752) construction
  line L394 (54.2644, -96.2752) -> (54.6956, -96.1282) construction
  line L395 (54.6956, -96.1282) -> (55.2406, -95.9466) construction
  line L396 (55.2406, -95.9466) -> (55.6729, -95.7395) construction
  line L397 (55.6729, -95.7395) -> (56.249, -95.3023) construction
  line L398 (56.249, -95.3023) -> (56.3816, -95.0223) construction
  line L399 (56.3816, -95.0223) -> (56.5338, -94.7522) construction
  line L400 (56.5338, -94.7522) -> (56.5044, -94.5704) construction
  line L401 (56.5044, -94.5704) -> (56.4258, -94.3396) construction
  line L402 (56.4258, -94.3396) -> (56.2932, -94.1971) construction
  line L403 (56.2932, -94.1971) -> (56.0132, -93.9515) construction
  line L404 (56.0132, -93.9515) -> (55.8462, -93.868) construction
  line L405 (55.8462, -93.868) -> (55.7578, -93.868) construction
  line L406 (55.7578, -93.868) -> (55.7234, -93.8337) construction
  line L407 (55.7234, -93.8337) -> (55.8855, -94.0203) construction
  line L408 (55.8855, -94.0203) -> (56.0672, -94.3248) construction
  line L409 (56.0672, -94.3248) -> (56.1311, -94.5704) construction
  line L410 (56.1311, -94.5704) -> (56.1311, -94.875) construction
  line L411 (56.1311, -94.875) -> (55.9395, -95.0862) construction
  line L412 (55.9395, -95.0862) -> (55.5711, -95.3367) construction
  line L413 (55.5711, -95.3367) -> (54.7558, -95.7492) construction
  line L414 (54.7558, -95.7492) -> (54.0239, -95.9801) construction
  line L415 (54.0239, -95.9801) -> (53.1363, -96.1078) construction
  line L416 (53.1363, -96.1078) -> (52.3441, -96.1078) construction
  line L417 (52.3441, -96.1078) -> (52.0494, -95.9997) construction
  line L418 (52.0494, -95.9997) -> (51.9168, -95.8917) construction
  line L419 (51.9168, -95.8917) -> (51.9168, -95.8327) construction
  line L420 (51.9168, -95.8327) -> (51.9525, -95.8597) construction
  line L421 (51.9525, -95.8597) -> (52.0734, -95.8176) construction
  line L422 (52.0734, -95.8176) -> (52.2438, -95.7451) construction
  line L423 (52.2438, -95.7451) -> (52.3617, -95.6893) construction
  line L424 (52.3617, -95.6893) -> (52.4405, -95.6346) construction
  line L425 (52.4405, -95.6346) -> (52.45, -95.6146) construction
  line L426 (52.45, -95.6146) -> (52.4269, -95.6146) construction
  line L427 (52.4269, -95.6146) -> (51.7074, -95.6241) construction
  line L428 (51.7074, -95.6241) -> (51.7074, -95.601) construction
  line L429 (51.7074, -95.601) -> (51.7558, -95.5557) construction
  line L430 (51.7558, -95.5557) -> (51.9041, -95.4484) construction
  line L431 (51.9041, -95.4484) -> (52.2661, -95.1189) construction
  line L432 (52.2661, -95.1189) -> (52.4745, -94.9137) construction
  line L433 (52.4745, -94.9137) -> (52.621, -94.7672) construction
  line L434 (52.621, -94.7672) -> (52.7057, -94.422) construction
  line L435 (52.7057, -94.422) -> (52.8164, -94.0964) construction
  line L436 (52.8164, -94.0964) -> (52.9239, -93.8848) construction
  line L437 (52.9239, -93.8848) -> (53.0606, -93.6959) construction
  line L438 (53.0606, -93.6959) -> (53.1363, -93.5716) construction
  spline S3 degree 4 poles (53.1363, -93.5716) (53.0988, -93.4618) (53.0207, -93.4126) (52.9369, -93.4762) (52.8039, -93.6352) (52.6092, -93.9366) (52.4824, -94.2341) (52.3511, -94.4615) (52.1762, -94.6759) (51.9637, -94.861) (51.6855, -95.0876) (51.4504, -95.3858) (51.3749, -95.5766) (51.3749, -95.7118) (51.3967, -95.8767) (51.6012, -96.1247) (51.9532, -96.3155) (52.3429, -96.4499) (52.9798, -96.4714) (53.3775, -96.4956) (53.7995, -96.4015) (54.2644, -96.2752) (54.6956, -96.1282) (55.2406, -95.9466) (55.6729, -95.7395) (56.249, -95.3023) (56.3816, -95.0223) (56.5338, -94.7522) (56.5044, -94.5704) (56.4258, -94.3396) (56.2932, -94.1971) (56.0132, -93.9515) (55.8462, -93.868) (55.7578, -93.868) (55.7234, -93.8337) (55.8855, -94.0203) (56.0672, -94.3248) (56.1311, -94.5704) (56.1311, -94.875) (55.9395, -95.0862) (55.5711, -95.3367) (54.7558, -95.7492) (54.0239, -95.9801) (53.1363, -96.1078) (52.3441, -96.1078) (52.0494, -95.9997) (51.9168, -95.8917) (51.9168, -95.8327) (51.9525, -95.8597) (52.0734, -95.8176) (52.2438, -95.7451) (52.3617, -95.6893) (52.4405, -95.6346) (52.45, -95.6146) (52.4269, -95.6146) (51.7074, -95.6241) (51.7074, -95.601) (51.7558, -95.5557) (51.9041, -95.4484) (52.2661, -95.1189) (52.4745, -94.9137) (52.621, -94.7672) (52.7057, -94.422) (52.8164, -94.0964) (52.9239, -93.8848) (53.0606, -93.6959) (53.1363, -93.5716) knots 1 1 1 1 1 2 3 4 5 6 7 8 9 10 11 12 13 14 15 16 17 18 19 20 21 22 23 24 25 26 27 28 29 30 31 32 33 34 35 36 37 38 39 40 41 42 43 44 45 46 47 48 49 50 51 52 53 54 55 56 57 58 59 60 61 62 63 64 64 64 64 64
  line L439 (53.4931, -94.0349) -> (53.9572, -94.0349) construction
  line L440 (53.9572, -94.0349) -> (54.2719, -93.9956) construction
  line L441 (54.2719, -93.9956) -> (54.5433, -93.8658) construction
  line L442 (54.5433, -93.8658) -> (54.7124, -93.7989) construction
  line L443 (54.7124, -93.7989) -> (54.9051, -93.7124) construction
  line L444 (54.9051, -93.7124) -> (54.8661, -93.8743) construction
  line L445 (54.8661, -93.8743) -> (54.7151, -94.1115) construction
  line L446 (54.7151, -94.1115) -> (54.4779, -94.3056) construction
  line L447 (54.4779, -94.3056) -> (54.176, -94.5069) construction
  line L448 (54.176, -94.5069) -> (53.9675, -94.5644) construction
  line L449 (53.9675, -94.5644) -> (53.7806, -94.5069) construction
  line L450 (53.7806, -94.5069) -> (53.6081, -94.3703) construction
  line L451 (53.6081, -94.3703) -> (53.4931, -94.1906) construction
  line L452 (53.4931, -94.1906) -> (53.4931, -94.0349) construction
  spline S4 degree 4 poles (53.4931, -94.0349) (53.9572, -94.0349) (54.2719, -93.9956) (54.5433, -93.8658) (54.7124, -93.7989) (54.9051, -93.7124) (54.8661, -93.8743) (54.7151, -94.1115) (54.4779, -94.3056) (54.176, -94.5069) (53.9675, -94.5644) (53.7806, -94.5069) (53.6081, -94.3703) (53.4931, -94.1906) (53.4931, -94.0349) knots 1 1 1 1 1 2 3 4 5 6 7 8 9 10 11 12 12 12 12 12
  line L453 (59.7761, -96.0245) -> (58.4894, -97.342) construction
  line L454 (58.4894, -97.342) -> (58.3202, -97.4291) construction
  line L455 (58.3202, -97.4291) -> (58.1972, -97.465) construction
  line L456 (58.1972, -97.465) -> (57.3051, -97.9213) construction
  line L457 (57.3051, -97.9213) -> (56.8899, -98.0187) construction
  line L458 (56.8899, -98.0187) -> (56.8284, -98.1161) construction
  line L459 (56.8284, -98.1161) -> (56.9773, -98.1161) construction
  line L460 (56.9773, -98.1161) -> (57.4411, -97.9786) construction
  line L461 (57.4411, -97.9786) -> (58.2055, -97.7173) construction
  line L462 (58.2055, -97.7173) -> (58.6105, -97.567) construction
  line L463 (58.6105, -97.567) -> (58.6634, -97.567) construction
  line L464 (58.6634, -97.567) -> (59.1013, -97.1509) construction
  line L465 (59.1013, -97.1509) -> (59.5511, -96.6814) construction
  line L466 (59.5511, -96.6814) -> (59.701, -96.4368) construction
  line L467 (59.701, -96.4368) -> (59.7997, -96.1882) construction
  line L468 (59.7997, -96.1882) -> (59.7761, -96.0245) construction
  spline S5 degree 4 poles (59.7761, -96.0245) (58.4894, -97.342) (58.3202, -97.4291) (58.1972, -97.465) (57.3051, -97.9213) (56.8899, -98.0187) (56.8284, -98.1161) (56.9773, -98.1161) (57.4411, -97.9786) (58.2055, -97.7173) (58.6105, -97.567) (58.6634, -97.567) (59.1013, -97.1509) (59.5511, -96.6814) (59.701, -96.4368) (59.7997, -96.1882) (59.7761, -96.0245) knots 1 1 1 1 1 2 3 4 5 6 7 8 9 10 11 12 13 14 14 14 14 14
  line L469 (61.1724, -95.6078) -> (62.7459, -96.1999) construction
  line L470 (62.7459, -96.1999) -> (62.786, -96.228) construction
  line L471 (62.786, -96.228) -> (62.8422, -96.228) construction
  line L472 (62.8422, -96.228) -> (63.3191, -96.228) construction
  line L473 (63.3191, -96.228) -> (64.3058, -96.228) construction
  line L474 (64.3058, -96.228) -> (64.3373, -96.2108) construction
  line L475 (64.3373, -96.2108) -> (64.7113, -96.0672) construction
  line L476 (64.7113, -96.0672) -> (65.5665, -95.7474) construction
  line L477 (65.5665, -95.7474) -> (65.5665, -95.6709) construction
  line L478 (65.5665, -95.6709) -> (65.4761, -95.6709) construction
  line L479 (65.4761, -95.6709) -> (65.344, -95.6709) construction
  line L480 (65.344, -95.6709) -> (64.6071, -95.949) construction
  line L481 (64.6071, -95.949) -> (64.1482, -96.0742) construction
  line L482 (64.1482, -96.0742) -> (63.5989, -96.0742) construction
  line L483 (63.5989, -96.0742) -> (62.8481, -96.0742) construction
  line L484 (62.8481, -96.0742) -> (62.5908, -95.9004) construction
  line L485 (62.5908, -95.9004) -> (61.9373, -95.7613) construction
  line L486 (61.9373, -95.7613) -> (61.1724, -95.6078) construction
  spline S6 degree 4 poles (61.1724, -95.6078) (62.7459, -96.1999) (62.786, -96.228) (62.8422, -96.228) (63.3191, -96.228) (64.3058, -96.228) (64.3373, -96.2108) (64.7113, -96.0672) (65.5665, -95.7474) (65.5665, -95.6709) (65.4761, -95.6709) (65.344, -95.6709) (64.6071, -95.949) (64.1482, -96.0742) (63.5989, -96.0742) (62.8481, -96.0742) (62.5908, -95.9004) (61.9373, -95.7613) (61.1724, -95.6078) knots 1 1 1 1 1 2 3 4 5 6 7 8 9 10 11 12 13 14 15 16 16 16 16 16
  line L487 (70.4606, -93.4832) -> (71.6637, -94.3855) construction
  line L488 (71.6637, -94.3855) -> (72.0679, -94.9119) construction
  line L489 (72.0679, -94.9119) -> (72.6036, -95.4852) construction
  line L490 (72.6036, -95.4852) -> (72.6036, -95.6078) construction
  line L491 (72.6036, -95.6078) -> (73.7014, -97.389) construction
  line L492 (73.7014, -97.389) -> (73.7885, -97.389) construction
  line L493 (73.7885, -97.389) -> (73.7416, -97.2147) construction
  line L494 (73.7416, -97.2147) -> (72.716, -95.2037) construction
  line L495 (72.716, -95.2037) -> (72.0591, -94.1982) construction
  line L496 (72.0591, -94.1982) -> (71.9853, -94.1513) construction
  line L497 (71.9853, -94.1513) -> (71.563, -93.9636) construction
  line L498 (71.563, -93.9636) -> (70.4606, -93.4832) construction